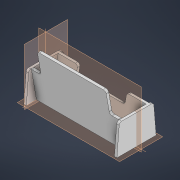
# Autodesk Inventor part: business card holder lgcc
Saved by Autodesk Inventor 2021 (Build 250183000, 183)
## iProperties
Created: 2020-08-19
Part Number: business card holder lgcc
Material: Generic
Document SubType Name: Modeling
Designer: brand
Density: 1 g/cm^3
Appearance: Default
Author: brand
Autodesk Inventor part; units mm, degrees
sketch "Sketch2" plane through (0, 0, 0) normal (1, 0, 0) x (0, 1, 0)
  line L0 (0, 20) -> (0, -20)
  line L1 (0, -20) -> (30, -17.5)
  line L2 (30, -17.5) -> (30, 17.5)
  line L3 (30, 17.5) -> (0, 20)
  line L4 (0, 28) -> (0, -28) projected
  line L5 (0, -28) -> (0, 28) projected
  line L6 (-6, 0) -> (36, 0) projected
  point P0 (0, 0)
  dimension "d4" = 30
  dimension "d5" = 35
  dimension "d6" = 40
  constraints: 8 end point, 2 parallel, 1 collinear, 1 vertical, 1 other
  measures "d4" distance between parallel lines of L0 L2
  measures "d5" distance of L1.end L2.end
  measures "d6" distance of L0.start L0.end
extrude "Extrusion1" add sketch "Sketch2" against normal blind 2.5
sketch "Sketch5" plane through (0, 0, 0) normal (1, 0, 0) x (0, 0, -1)
  line L0 (-17.5, 30) -> (17.5, 30) projected
  line L1 (15, 30) -> (9.7102, 0)
  line L2 (9.7102, 0) -> (-9.6716, 0)
  line L3 (-9.6716, 0) -> (-18.8522, 52.0659)
  line L4 (-18.8522, 52.0659) -> (-16.3902, 52.5)
  line L5 (-16.3902, 52.5) -> (-7.5739, 2.5)
  line L6 (-7.5739, 2.5) -> (7.6124, 2.5)
  line L7 (7.6124, 2.5) -> (12.4614, 30)
  line L8 (12.4614, 30) -> (15, 30)
  line L9 (-20, 0) -> (20, 0) projected
  point P0 (0, 0)
  dimension "d15" = 2.5
  dimension "d16" = 2.5
  dimension "d17" = 2.5
  dimension "d18" = 2.5
  dimension "d19" = 2.5
  dimension "d20" = 50
  dimension "d22" = 100
  dimension "d23" = 100
  constraints: 16 end point, 4 parallel, 2 perpendicular, 1 collinear, 1 point on line
  measures "d15" distance between parallel lines of L1 L7
  measures "d16" distance between parallel lines of L2 L6
  measures "d17" distance between parallel lines of L5 L3
  measures "d18" distance of L0.end L1.start
  measures "d19" distance from line of L3 L0.start
  measures "d20" vertical distance of L4.end L5.end
  measures "d22" angle of L6 L5
  measures "d23" angle of L6 L7
extrude "Extrusion2" add sketch "Sketch5" along normal blind 45 contours L0 L1 L2 L3 L5 L6 L7 | L0 L3 L4 L5
sketch "Sketch8" plane through (45, 30, -15) normal (0, -0.1736482, -0.9848078) x (-1, 0, 0)
  line L0 (0, 0) -> (25, 0)
  line L1 (25, 0) -> (25, -10)
  line L2 (25, -10) -> (0, -10)
  line L3 (0, -10) -> (0, 0)
  line L4 (45, 0) -> (0, 0) projected
  point P0 (45, -32.149)
  dimension "d33" = 10
  dimension "d34" = 25
  constraints: 8 end point, 2 parallel, 1 collinear, 1 horizontal, 1 perpendicular
  measures "d33" distance between parallel lines of L0 L2
  measures "d34" distance between parallel lines of L3 L1
extrude "Extrusion5" cut sketch "Sketch8" against normal blind 2.5
sketch "Sketch9" plane through (45, 52.5, 16.3902) normal (0, 0.1736482, -0.9848078) x (-1, 0, 0)
  line L0 (45, 0) -> (45, -22.4063) projected
  line L1 (45, 0) -> (35, 0)
  line L2 (35, 0) -> (35, -22.8471)
  line L3 (35, -22.8471) -> (45, -22.8471)
  line L4 (45, -22.8471) -> (45, 0)
  point P0 (45, -54.5485)
  point P1 (45, -20)
  point P2 (45, -22.4063)
  dimension "d38" = 10
  constraints: 8 end point, 2 parallel, 1 horizontal, 1 perpendicular, 1 point on line
  measures "d38" distance of L2.end L3.end
extrude "Extrusion6" cut sketch "Sketch9" against normal blind 2.5
fillet "Fillet1" radius 2.5 7 edges at (10, 52.2829, 17.6212) (10, 29.7829, 13.6539) (-1.25, 30, 17.5) (-1.25, 30, -17.5) (20, 30, -13.7307) (20, 20.369, -12.0325) (0, 29.7829, 13.6539)
mirror "Mirror1" about plane through (45, 26.25, 1.9261) normal (1, 0, 0)
equation "\"d15\" = thickness"
equation "\"d16\" = thickness"
equation "\"d17\" = thickness"
equation "\"d18\" = thickness"
equation "\"d19\" = thickness"
equation "\"d22\" = d23"
equation "\"d35\" = thickness"
equation "\"d39\" = thickness"
equation "\"thickness\" = 2.5"
body "Solid1"
